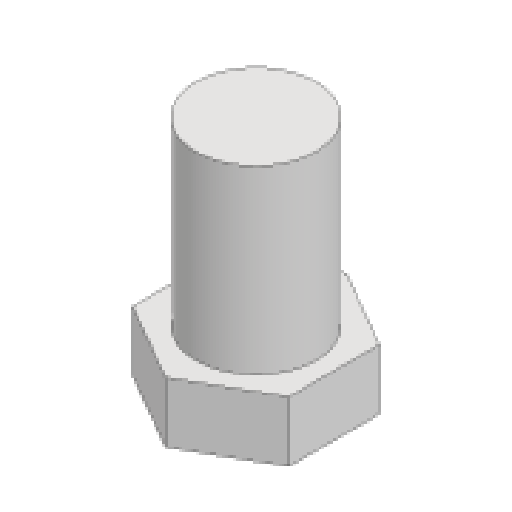
# Autodesk Inventor part: M4 bolt
Saved by Autodesk Inventor 2023 (Build 270158000, 158)
## iProperties
Created: 2022-09-21
Part Number: M4 bolt
Material: Generic
Document SubType Name: Modeling
Designer: CDT
Density: 1 g/cm^3
Appearance: Default
Author: CDT
Autodesk Inventor part; units mm, degrees
ref_plane "YZ Plane" through (0, 0, 0) normal (1, 0, 0) x (0, 1, 0)
ref_plane "XZ Plane" through (0, 0, 0) normal (0, 1, 0) x (-1, 0, 0)
ref_plane "XY Plane" through (0, 0, 0) normal (0, 0, 1) x (1, 0, 0)
sketch "Sketch1" plane through (0, 0, 0) normal (0, 1, 0) x (-1, 0, 0)
  line L0 (0, -3) -> (-2.5981, -1.5)
  line L1 (-2.5981, -1.5) -> (-2.5981, 1.5)
  line L2 (-2.5981, 1.5) -> (0, 3)
  line L3 (0, 3) -> (2.5981, 1.5)
  line L4 (2.5981, 1.5) -> (2.5981, -1.5)
  line L5 (2.5981, -1.5) -> (0, -3)
  point P0 (0, 0)
  point P1 (0, 0)
  dimension "d5" = 6
  constraints: 12 end point, 1 coincident, 13 other
  measures "d5" distance of L0.start L2.end
extrude "Extrusion1" add sketch "Sketch1" along normal blind 2
sketch "Sketch2" plane through (0, 2, 0) normal (0, 1, 0) x (1, 0, 0)
  circle A0 centre (0, 0) radius 2
  dimension "d2" = 4
  constraints: 1 centre point, 1 coincident
  measures "d2" diameter of A0
extrude "Extrusion2" add sketch "Sketch2" along normal blind 10
thread "Thread1" size "M4x0.7" class "6g" standard "ANSI Metric M Profile" full length
body "Solid1"
